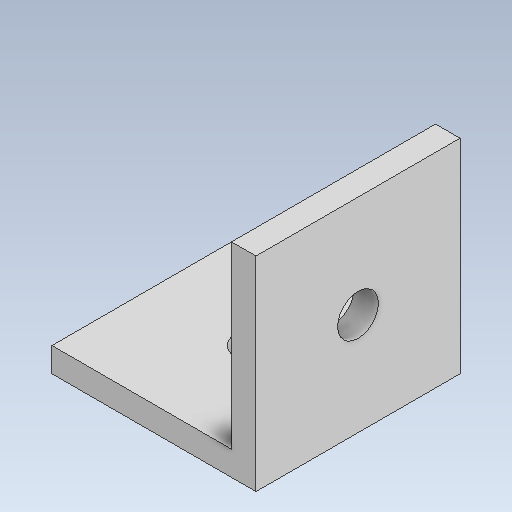
# Autodesk Inventor part: WCDLBRACKET
Saved by Autodesk Inventor 2020 (Build 240168000, 168)
## iProperties
Created: 2021-01-19
Part Number: WCDLBRACKET
Material: Generic
Document SubType Name: Modeling
Designer: lucky
Density: 1 g/cm^3
Appearance: Default
Mass: 3.40719 g
Surface Area: 27.9771 cm^2
Volume: 3.40719 cm^3
Author: lucky
Autodesk Inventor part; units mm, degrees
ref_plane "YZ Plane" through (0, 0, 0) normal (1, 0, 0) x (0, 1, 0)
ref_plane "XZ Plane" through (0, 0, 0) normal (0, 1, 0) x (-1, 0, 0)
ref_plane "XY Plane" through (0, 0, 0) normal (0, 0, 1) x (1, 0, 0)
sketch "Sketch1" plane through (0, 0, 0) normal (0, 1, 0) x (-1, 0, 0)
  line L0 (-12.5, 12.5) -> (12.5, 12.5)
  line L1 (12.5, 12.5) -> (12.5, -12.5)
  line L2 (12.5, -12.5) -> (-12.5, -12.5)
  line L3 (-12.5, -12.5) -> (-12.5, 12.5)
  line L4 (-12.5, 12.5) -> (12.5, -12.5) construction
  line L5 (12.5, 12.5) -> (-12.5, -12.5) construction
  point P0 (0, 0)
  dimension "d0" = 25
  dimension "d1" = 25
  constraints: 12 end point, 2 midpoint, 2 parallel, 1 horizontal, 1 perpendicular
  measures "d0" distance of L1.end L2.end
  measures "d1" distance of L0.end L1.end
extrude "Extrusion1" add sketch "Sketch1" along normal mid plane 3
sketch "Sketch2" plane through (0, 1.5, 0) normal (0, 1, 0) x (1, 0, 0)
  line L0 (12.5, -12.5) -> (12.5, 12.5) projected
  line L1 (12.5, 12.5) -> (-12.5, 12.5) projected
  line L2 (12.5, -12.5) -> (9.5, -12.5)
  line L3 (9.5, -12.5) -> (9.5, 12.5)
  line L4 (9.5, 12.5) -> (12.5, 12.5)
  line L5 (12.5, 12.5) -> (12.5, -12.5)
  point P0 (0, 0)
  dimension "d4" = 3
  constraints: 8 end point, 2 parallel, 1 horizontal, 1 perpendicular, 1 point on line
  measures "d4" distance between parallel lines of L0 L3
extrude "Extrusion2" add sketch "Sketch2" along normal blind 22
sketch "Sketch3" plane through (12.5, -1.5, 12.5) normal (1, 0, 0) x (0, 0, -1)
  line L0 (25, 0) -> (25, 25) projected
  line L1 (25, 0) -> (0, 0) projected
  point P0 (12.5, 1.5)
  point P1 (12.5, 12.5)
  point P2 (25, 12.5)
  point P3 (12.5, 0)
  constraints: 2 midpoint, 1 horizontal alignment, 1 vertical alignment
hole "Hole1" at (12.5, 11, 0) direction (-1, 0, 0) diameter 5 end through all
sketch "Sketch4" plane through (0, -1.5, 0) normal (0, -1, 0) x (1, 0, 0)
  point P0 (0, 0)
  point P1 (0, 0)
  constraints: 1 coincident
hole "Hole2" at (0, -1.5, 0) direction (0, 1, 0) diameter 5 end through all
body "Solid1"
